Flystop Anchor (Autodesk Fusion 360 design; units mm, degrees)
Autodesk Fusion 360 part; units mm, degrees
note: some values were not read from the file. Set by a fixed rule: which sketch regions a step uses.
sketch "Sketch2" plane through (0, 0, 0) normal (0, 0, 1) x (1, 0, 0)
  line L0 (0, 0) -> (-2, 0)
  line L1 (-2, 0) -> (-2, 32)
  line L2 (-2, 32) -> (0, 32)
  line L3 (0, 32) -> (0, 0)
  line L4 (-2, 0) -> (18, 0)
  line L5 (18, 0) -> (18, -2)
  line L6 (18, -2) -> (-2, -2)
  line L7 (-2, -2) -> (-2, 0)
  line L8 (18, 0) -> (20, 0)
  line L9 (20, 0) -> (20, -14)
  line L10 (20, -14) -> (18, -14)
  line L11 (18, -14) -> (18, 0)
  dimension "d5" = 2
  dimension "d6" = 32
  dimension "d7" = 20
  dimension "d8" = 2
  dimension "d9" = 2
  dimension "d10" = 14
  constraint horizontal L0
  constraint vertical L1
  constraint horizontal L2
  constraint vertical L3
  constraint coincident L0.start L3.end
  constraint horizontal L4
  constraint vertical L5
  constraint horizontal L6
  constraint vertical L7
  constraint horizontal L8
  constraint vertical L9
  constraint horizontal L10
  constraint vertical L11
  measures "d5" distance of L0.start L0.end
  measures "d6" distance of L0.start L2.end
  measures "d7" distance of L0.end L4.end
  measures "d8" distance of L0.end L6.end
  measures "d9" distance of L4.end L8.end
  measures "d10" distance of L4.end L10.end
extrude "Extrude1" add sketch "Sketch2" along normal blind 10
sketch "Sketch3" plane through (0, 0, 0) normal (1, 0, 0) x (0, 1, 0)
  line L0 (0, 0) -> (32, 0)
  line L1 (32, 0) -> (32, 10)
  line L2 (32, 10) -> (0, 10)
  line L3 (0, 10) -> (0, 0)
  circle A0 centre (27, 5) radius 1
  circle A1 centre (15, 5) radius 1
  circle A2 centre (5, 5) radius 1
  line L4 (5, 6) -> (15, 6)
  line L5 (15, 6) -> (15, 4)
  line L6 (15, 4) -> (5, 4)
  line L7 (5, 4) -> (5, 6)
  dimension "d15" = 2
  dimension "d16" = 5
  dimension "d17" = 5
  dimension "d18" = 2
  dimension "d19" = 15
  dimension "d20" = 2
  dimension "d21" = 5
  dimension "d22" = 5
  dimension "d23" = 5
  dimension "d24" = 2
  constraint horizontal L4
  constraint vertical L5
  constraint horizontal L6
  constraint vertical L7
  constraint coincident A2.centre L7
  constraint coincident A1.centre L5
  constraint tangent A2 L4
  measures "d15" diameter of A0
  measures "d16" distance of L1 A0.centre
  measures "d17" distance of L2 A0.centre
  measures "d18" diameter of A1
  measures "d19" distance of L3 A1.centre
  measures "d20" diameter of A2
  measures "d21" distance of L2 A1.centre
  measures "d22" distance of L2 A2.centre
  measures "d23" distance of L3 A2.centre
  measures "d24" distance of L4.start L6.end
extrude "Extrude2" cut sketch "Sketch3" against normal blind 2 contours A0 | A1 L5 | A1 L5 | A1 A2 L4 L6 | A2 L7 | A2 L7
fillet "Fillet1" radius 2 1 edges at (0, 0, 5)
fillet "Fillet1" radius 2 1 edges at (18, -2, 5)
fillet "Fillet1" radius 1 1 edges at (20, 0, 5)
equation "thickness = 2 mm"
equation "d5 = thickness"
equation "d7 = window_depth"
equation "d8 = thickness"
equation "d9 = thickness"
equation "width = 10 mm"
equation "d12 = width"
equation "hole = 2 mm"
equation "d15 = hole"
equation "d16 = width / 2"
equation "d17 = width / 2"
equation "d18 = hole"
equation "d19 = width + width / 2"
equation "d20 = hole"
equation "d21 = width / 2"
equation "d22 = width / 2"
equation "d23 = width / 2"
equation "d24 = hole"
equation "d25 = -thickness"
equation "d28 = thickness"
equation "d30 = thickness"
equation "d32 = thickness / 2"
equation "window_depth = 20 mm"
